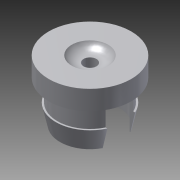
# Autodesk Inventor part: Cable end barrel stop
Saved by Autodesk Inventor 2014 SP2 (Build 180246200, 246)
## iProperties
Created: 2014-08-06
Part Number: Cable end barrel stop
Material: PC/ABS Plastic
Document SubType Name: Modeling
Designer: Lukasz Szmit
Density: 0.357273 g/cm^3
Appearance: Smooth - White
Author: Lukasz Szmit
Autodesk Inventor part; units mm, degrees
ref_plane "XZ Plane" through (0, 0, 0) normal (0, 1, 0) x (-1, 0, 0)
ref_plane "XY Plane" through (0, 0, 0) normal (0, 0, 1) x (1, 0, 0)
sketch "Sketch1" plane through (0, 0, 0) normal (0, 0, 1) x (1, 0, 0)
  circle A0 centre (0, 0) radius 6.4
  dimension "d0" = 12.8
  constraints: 1 centre point, 1 coincident
  measures "d0" diameter of A0
sketch "Sketch2" plane through (0, 0, 0) normal (0, 0, 1) x (1, 0, 0)
  circle A0 centre (0, 0) radius 2.825
  dimension "d3" = 5.65
  constraints: 1 centre point, 1 coincident
  measures "d3" diameter of A0
sketch "Sketch3" plane through (0, 0, 0) normal (0, 0, 1) x (1, 0, 0)
  circle A0 centre (0, 0) radius 1
  dimension "d4" = 2
  constraints: 1 centre point, 1 coincident
  measures "d4" diameter of A0
extrude "Extrusion1" add sketch "Sketch1" against normal blind 3
extrude "Extrusion2" cut sketch "Sketch2" against normal blind 1
extrude "Extrusion3" cut sketch "Sketch3" against normal blind 3
fillet "Fillet1" radius 2 1 edges at (-2.825, 0, -1)
sketch "Sketch4" plane through (0, 0, 0) normal (0, 1, 0) x (-1, 0, 0)
  line L0 (-5.0465, -3) -> (-5.0465, -6.35)
  line L1 (-6.4, -3) -> (6.4, -3) projected
  line L2 (-5.2965, -6.35) -> (-5.0465, -6.35)
  line L3 (-4.5465, -4) -> (-4.5465, -9.35)
  line L4 (0, -3) -> (0, -11.7949)
  arc A0 (-3.5465, -3) -> (-4.5465, -4) centre (-3.5465, -4) ccw
  line L5 (-5.0465, -3) -> (-3.5465, -3)
  line L6 (-4.5465, -9.35) -> (-4.6465, -9.35)
  line L7 (-4.6465, -9.35) -> (-5.2965, -6.35)
  point P0 (0, 0)
  point P1 (-4.5465, -3)
  dimension "d21" = 0.25
  dimension "d26" = 6.35
  dimension "d28" = 0.5
  dimension "d29" = 90
  dimension "d40" = 1
  dimension "d41" = 3
  dimension "d42" = 0.1
  constraints: 14 end point, 2 perpendicular, 2 point on circle, 2 point on line, 1 centre point, 1 midpoint, 1 parallel, 1 tangent
  measures "d21" distance from line of L0 L2.start
  measures "d26" distance of point (-4.546, -3) L3.end
  measures "d28" distance between parallel lines of L0 L3
  measures "d29" angle of L0 L2
  measures "d40" radius of A0
  measures "d41" vertical distance of L6.end L2.start
  measures "d42" distance of L3.end L6.end
revolve "Revolution2" add sketch "Sketch4" angle 360 about axis through (0, 0, -3) along (0, 0, -1)
ref_plane "Work Plane2" through (6.4, 0, 0) normal (1, 0, 0) x (0, 1, 0)
sketch "Sketch7" plane through (6.4, 0, 0) normal (1, 0, 0) x (0, 1, 0)
  line L0 (-2.15, -3) -> (-2.15, -9.35)
  line L1 (-2.15, -9.35) -> (2.15, -9.35)
  line L2 (2.15, -9.35) -> (2.15, -3)
  line L3 (2.15, -3) -> (-2.15, -3)
  point P0 (0, 0)
  dimension "d34" = 4.3
  dimension "d35" = 6.35
  constraints: 8 end point, 2 parallel, 1 perpendicular
  measures "d34" distance of L2.end L0.start
  measures "d35" distance of L0.start L0.end
extrude "Extrusion4" cut sketch "Sketch7" against normal blind 12.8
fillet "Fillet3" radius 1 4 edges at (3.693, -2.15, -3) (-3.693, -2.15, -3) (-3.693, 2.15, -3) (3.693, 2.15, -3)
body "Solid1"
